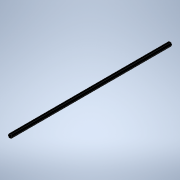
# Autodesk Inventor part: Hex Shaft
Saved by Autodesk Inventor 2020 (Build 240168000, 168)
## iProperties
Created: 2020-01-26
Part Number: Hex Shaft
Material: Aluminum 6061
Document SubType Name: Modeling
Designer: autum
Density: 2.7 g/cm^3
Appearance: Anodized - Black
Author: autum
Autodesk Inventor part; units mm, degrees
ref_plane "YZ Plane" through (0, 0, 0) normal (1, 0, 0) x (0, 1, 0)
ref_plane "XZ Plane" through (0, 0, 0) normal (0, 1, 0) x (-1, 0, 0)
ref_plane "XY Plane" through (0, 0, 0) normal (0, 0, 1) x (1, 0, 0)
sketch "Sketch1" plane through (0, 0, 0) normal (0, 0, 1) x (1, 0, 0)
  line L0 (6.35, 0) -> (3.175, -5.4993)
  line L1 (3.175, -5.4993) -> (-3.175, -5.4993)
  line L2 (-3.175, -5.4993) -> (-6.35, 0)
  line L3 (-6.35, 0) -> (-3.175, 5.4993)
  line L4 (-3.175, 5.4993) -> (3.175, 5.4993)
  line L5 (3.175, 5.4993) -> (6.35, 0)
  point P0 (0, 0)
  point P1 (0, 0)
  dimension "d0" = 12.7
  constraints: 12 end point, 1 coincident, 13 other
  measures "d0" distance of L0.start L2.end
extrude "Extrusion1" add sketch "Sketch1" along normal blind 508
body "Solid1"
